Autodesk Fusion 360 part; units mm, degrees
(part 4 of 18)
  line L2686 (171.4183, -55.0432) -> (170.8263, -55.4974)
  line L2687 (174.8684, -55.4974) -> (174.2764, -55.0432)
  line L2688 (173.5871, -54.7577) -> (172.8473, -54.6603)
  line L2689 (174.2764, -55.0432) -> (173.5871, -54.7577)
  line L2690 (172.1076, -54.7577) -> (171.4183, -55.0432)
  line L2691 (170.3721, -58.9475) -> (170.8263, -59.5394)
  line L2692 (175.7055, -57.5184) -> (175.6081, -56.7787)
  line L2693 (175.6081, -56.7787) -> (175.3226, -56.0893)
  line L2694 (174.8684, -59.5394) -> (175.3226, -58.9475)
  line L2695 (172.8473, -54.6603) -> (172.1076, -54.7577)
  line L2696 (175.3226, -58.9475) -> (175.6081, -58.2582)
  line L2697 (170.0866, -58.2582) -> (170.3721, -58.9475)
  line L2698 (172.3659, -83.7435) -> (172.8473, -83.8393)
  line L2699 (173.737, -81.6915) -> (173.3288, -81.4188)
  line L2700 (173.3288, -81.4188) -> (172.8473, -81.323)
  line L2701 (173.3288, -83.7435) -> (173.737, -83.4708)
  line L2702 (173.737, -83.4708) -> (174.0097, -83.0626)
  line L2703 (172.8473, -81.323) -> (172.3659, -81.4188)
  line L2704 (171.9577, -83.4708) -> (172.3659, -83.7435)
  line L2705 (174.0097, -83.0626) -> (174.1055, -82.5812)
  line L2706 (172.3659, -81.4188) -> (171.9577, -81.6915)
  line L2707 (174.1055, -82.5812) -> (174.0097, -82.0997)
  line L2708 (171.5892, -82.5812) -> (171.685, -83.0626)
  line L2709 (171.685, -82.0997) -> (171.5892, -82.5812)
  line L2710 (172.8473, -83.8393) -> (173.3288, -83.7435)
  line L2711 (171.9577, -81.6915) -> (171.685, -82.0997)
  line L2712 (171.685, -83.0626) -> (171.9577, -83.4708)
  line L2713 (174.0097, -82.0997) -> (173.737, -81.6915)
  line L2714 (172.3659, -64.6808) -> (172.8473, -64.7766)
  line L2715 (171.5892, -63.5184) -> (171.685, -63.9999)
  line L2716 (171.9577, -64.4081) -> (172.3659, -64.6808)
  line L2717 (174.0097, -63.9999) -> (174.1055, -63.5184)
  line L2718 (171.9577, -62.6288) -> (171.685, -63.037)
  line L2719 (173.737, -64.4081) -> (174.0097, -63.9999)
  line L2720 (172.8473, -62.2603) -> (172.3659, -62.3561)
  line L2721 (173.3288, -64.6808) -> (173.737, -64.4081)
  line L2722 (171.685, -63.9999) -> (171.9577, -64.4081)
  line L2723 (173.737, -62.6288) -> (173.3288, -62.3561)
  line L2724 (172.8473, -64.7766) -> (173.3288, -64.6808)
  line L2725 (171.685, -63.037) -> (171.5892, -63.5184)
  line L2726 (174.0097, -63.037) -> (173.737, -62.6288)
  line L2727 (172.3659, -62.3561) -> (171.9577, -62.6288)
  line L2728 (173.3288, -62.3561) -> (172.8473, -62.2603)
  line L2729 (174.1055, -63.5184) -> (174.0097, -63.037)
  line L2730 (174.1055, -25.4057) -> (174.0097, -24.9242)
  line L2731 (171.9577, -24.516) -> (171.685, -24.9242)
  line L2732 (173.737, -24.516) -> (173.3288, -24.2433)
  line L2733 (172.8473, -24.1475) -> (172.3659, -24.2433)
  line L2734 (171.5892, -25.4057) -> (171.685, -25.8871)
  line L2735 (173.737, -26.2953) -> (174.0097, -25.8871)
  line L2736 (174.0097, -25.8871) -> (174.1055, -25.4057)
  line L2737 (172.8473, -26.6638) -> (173.3288, -26.568)
  line L2738 (174.0097, -24.9242) -> (173.737, -24.516)
  line L2739 (173.3288, -26.568) -> (173.737, -26.2953)
  line L2740 (171.9577, -26.2953) -> (172.3659, -26.568)
  line L2741 (173.3288, -24.2433) -> (172.8473, -24.1475)
  line L2742 (172.3659, -26.568) -> (172.8473, -26.6638)
  line L2743 (171.685, -24.9242) -> (171.5892, -25.4057)
  line L2744 (171.685, -25.8871) -> (171.9577, -26.2953)
  line L2745 (172.3659, -24.2433) -> (171.9577, -24.516)
  line L2746 (171.9577, -45.3453) -> (172.3659, -45.6181)
  line L2747 (174.1055, -44.4557) -> (174.0097, -43.9742)
  line L2748 (174.0097, -44.9372) -> (174.1055, -44.4557)
  line L2749 (173.3288, -43.2933) -> (172.8473, -43.1975)
  line L2750 (173.737, -43.566) -> (173.3288, -43.2933)
  line L2751 (173.737, -45.3453) -> (174.0097, -44.9372)
  line L2752 (172.8473, -43.1975) -> (172.3659, -43.2933)
  line L2753 (172.8473, -45.7138) -> (173.3288, -45.6181)
  line L2754 (171.685, -43.9742) -> (171.5892, -44.4557)
  line L2755 (173.3288, -45.6181) -> (173.737, -45.3453)
  line L2756 (172.3659, -43.2933) -> (171.9577, -43.566)
  line L2757 (172.3659, -45.6181) -> (172.8473, -45.7138)
  line L2758 (171.9577, -43.566) -> (171.685, -43.9742)
  line L2759 (174.0097, -43.9742) -> (173.737, -43.566)
  line L2760 (171.685, -44.9372) -> (171.9577, -45.3453)
  line L2761 (171.5892, -44.4557) -> (171.685, -44.9372)
  line L2762 (189.8764, -21.4267) -> (190.4683, -21.8809)
  line L2763 (189.8764, -17.3846) -> (189.4222, -17.9766)
  line L2764 (189.4222, -20.8347) -> (189.8764, -21.4267)
  line L2765 (193.9184, -17.3846) -> (193.3265, -16.9304)
  line L2766 (191.8974, -16.5475) -> (191.1576, -16.6449)
  line L2767 (189.1366, -20.1454) -> (189.4222, -20.8347)
  line L2768 (191.8974, -22.2638) -> (192.6371, -22.1664)
  line L2769 (193.3265, -16.9304) -> (192.6371, -16.6449)
  line L2770 (194.3726, -17.9766) -> (193.9184, -17.3846)
  line L2771 (189.4222, -17.9766) -> (189.1366, -18.6659)
  line L2772 (194.6581, -18.6659) -> (194.3726, -17.9766)
  line L2773 (194.6581, -20.1454) -> (194.7555, -19.4056)
  line L2774 (193.9184, -21.4267) -> (194.3726, -20.8347)
  line L2775 (191.1576, -22.1664) -> (191.8974, -22.2638)
  line L2776 (194.3726, -20.8347) -> (194.6581, -20.1454)
  line L2777 (190.4683, -21.8809) -> (191.1576, -22.1664)
  line L2778 (193.3265, -21.8809) -> (193.9184, -21.4267)
  line L2779 (194.7555, -19.4056) -> (194.6581, -18.6659)
  line L2780 (190.4683, -16.9304) -> (189.8764, -17.3846)
  line L2781 (192.6371, -16.6449) -> (191.8974, -16.5475)
  line L2782 (191.1576, -16.6449) -> (190.4683, -16.9304)
  line L2783 (192.6371, -22.1664) -> (193.3265, -21.8809)
  line L2784 (189.1366, -18.6659) -> (189.0392, -19.4056)
  line L2785 (189.0392, -19.4056) -> (189.1366, -20.1454)
  line L2786 (189.4222, -78.0102) -> (189.8764, -78.6022)
  line L2787 (192.6371, -79.3419) -> (193.3265, -79.0564)
  line L2788 (192.6371, -73.8204) -> (191.8974, -73.723)
  line L2789 (193.3265, -74.1059) -> (192.6371, -73.8204)
  line L2790 (191.1576, -79.3419) -> (191.8974, -79.4393)
  line L2791 (194.6581, -75.8414) -> (194.3726, -75.1521)
  line L2792 (194.6581, -77.3209) -> (194.7555, -76.5812)
  line L2793 (190.4683, -74.1059) -> (189.8764, -74.5601)
  line L2794 (191.8974, -79.4393) -> (192.6371, -79.3419)
  line L2795 (191.8974, -73.723) -> (191.1576, -73.8204)
  line L2796 (189.1366, -75.8414) -> (189.0392, -76.5812)
  line L2797 (189.0392, -76.5812) -> (189.1366, -77.3209)
  line L2798 (194.7555, -76.5812) -> (194.6581, -75.8414)
  line L2799 (194.3726, -78.0102) -> (194.6581, -77.3209)
  line L2800 (189.1366, -77.3209) -> (189.4222, -78.0102)
  line L2801 (193.9184, -74.5601) -> (193.3265, -74.1059)
  line L2802 (193.3265, -79.0564) -> (193.9184, -78.6022)
  line L2803 (189.4222, -75.1521) -> (189.1366, -75.8414)
  line L2804 (190.4683, -79.0564) -> (191.1576, -79.3419)
  line L2805 (191.1576, -73.8204) -> (190.4683, -74.1059)
  line L2806 (189.8764, -78.6022) -> (190.4683, -79.0564)
  line L2807 (193.9184, -78.6022) -> (194.3726, -78.0102)
  line L2808 (194.3726, -75.1521) -> (193.9184, -74.5601)
  line L2809 (189.8764, -74.5601) -> (189.4222, -75.1521)
  line L2810 (194.7555, -38.4557) -> (194.6581, -37.7159)
  line L2811 (191.1576, -35.6949) -> (190.4683, -35.9805)
  line L2812 (189.1366, -39.1954) -> (189.4222, -39.8847)
  line L2813 (189.4222, -37.0266) -> (189.1366, -37.7159)
  line L2814 (193.9184, -36.4347) -> (193.3265, -35.9805)
  line L2815 (193.3265, -35.9805) -> (192.6371, -35.6949)
  line L2816 (194.6581, -37.7159) -> (194.3726, -37.0266)
  line L2817 (192.6371, -35.6949) -> (191.8974, -35.5975)
  line L2818 (189.1366, -37.7159) -> (189.0392, -38.4557)
  line L2819 (190.4683, -35.9805) -> (189.8764, -36.4347)
  line L2820 (189.8764, -36.4347) -> (189.4222, -37.0266)
  line L2821 (194.3726, -37.0266) -> (193.9184, -36.4347)
  line L2822 (189.8764, -40.4767) -> (190.4683, -40.9309)
  line L2823 (191.1576, -41.2164) -> (191.8974, -41.3138)
  line L2824 (190.4683, -40.9309) -> (191.1576, -41.2164)
  line L2825 (193.3265, -40.9309) -> (193.9184, -40.4767)
  line L2826 (193.9184, -40.4767) -> (194.3726, -39.8847)
  line L2827 (194.3726, -39.8847) -> (194.6581, -39.1954)
  line L2828 (191.8974, -41.3138) -> (192.6371, -41.2164)
  line L2829 (191.8974, -35.5975) -> (191.1576, -35.6949)
  line L2830 (194.6581, -39.1954) -> (194.7555, -38.4557)
  line L2831 (192.6371, -41.2164) -> (193.3265, -40.9309)
  line L2832 (189.0392, -38.4557) -> (189.1366, -39.1954)
  line L2833 (189.4222, -39.8847) -> (189.8764, -40.4767)
  line L2834 (189.1366, -58.2582) -> (189.4222, -58.9475)
  line L2835 (189.0392, -57.5184) -> (189.1366, -58.2582)
  line L2836 (190.4683, -55.0432) -> (189.8764, -55.4974)
  line L2837 (190.4683, -59.9936) -> (191.1576, -60.2792)
  line L2838 (191.1576, -54.7577) -> (190.4683, -55.0432)
  line L2839 (191.8974, -60.3766) -> (192.6371, -60.2792)
  line L2840 (192.6371, -54.7577) -> (191.8974, -54.6603)
  line L2841 (192.6371, -60.2792) -> (193.3265, -59.9936)
  line L2842 (191.8974, -54.6603) -> (191.1576, -54.7577)
  line L2843 (194.3726, -58.9475) -> (194.6581, -58.2582)
  line L2844 (189.1366, -56.7787) -> (189.0392, -57.5184)
  line L2845 (193.3265, -55.0432) -> (192.6371, -54.7577)
  line L2846 (191.1576, -60.2792) -> (191.8974, -60.3766)
  line L2847 (194.3726, -56.0893) -> (193.9184, -55.4974)
  line L2848 (189.4222, -58.9475) -> (189.8764, -59.5394)
  line L2849 (193.3265, -59.9936) -> (193.9184, -59.5394)
  line L2850 (189.4222, -56.0893) -> (189.1366, -56.7787)
  line L2851 (194.7555, -57.5184) -> (194.6581, -56.7787)
  line L2852 (189.8764, -59.5394) -> (190.4683, -59.9936)
  line L2853 (194.6581, -56.7787) -> (194.3726, -56.0893)
  line L2854 (189.8764, -55.4974) -> (189.4222, -56.0893)
  line L2855 (193.9184, -59.5394) -> (194.3726, -58.9475)
  line L2856 (193.9184, -55.4974) -> (193.3265, -55.0432)
  line L2857 (194.6581, -58.2582) -> (194.7555, -57.5184)
  line L2858 (193.0598, -82.0997) -> (192.787, -81.6915)
  line L2859 (193.0598, -83.0626) -> (193.1555, -82.5812)
  line L2860 (191.0077, -83.4708) -> (191.4159, -83.7435)
  line L2861 (191.8974, -81.323) -> (191.4159, -81.4188)
  line L2862 (192.3789, -83.7435) -> (192.787, -83.4708)
  line L2863 (192.3789, -81.4188) -> (191.8974, -81.323)
  line L2864 (191.4159, -81.4188) -> (191.0077, -81.6915)
  line L2865 (190.735, -82.0997) -> (190.6392, -82.5812)
  line L2866 (191.0077, -81.6915) -> (190.735, -82.0997)
  line L2867 (193.1555, -82.5812) -> (193.0598, -82.0997)
  line L2868 (192.787, -81.6915) -> (192.3789, -81.4188)
  line L2869 (192.787, -83.4708) -> (193.0598, -83.0626)
  line L2870 (191.8974, -83.8393) -> (192.3789, -83.7435)
  line L2871 (191.4159, -83.7435) -> (191.8974, -83.8393)
  line L2872 (190.6392, -82.5812) -> (190.735, -83.0626)
  line L2873 (190.735, -83.0626) -> (191.0077, -83.4708)
  line L2874 (192.3789, -64.6808) -> (192.787, -64.4081)
  line L2875 (192.3789, -62.3561) -> (191.8974, -62.2603)
  line L2876 (191.4159, -62.3561) -> (191.0077, -62.6288)
  line L2877 (190.735, -63.9999) -> (191.0077, -64.4081)
  line L2878 (193.0598, -63.9999) -> (193.1555, -63.5184)
  line L2879 (191.4159, -64.6808) -> (191.8974, -64.7766)
  line L2880 (192.787, -62.6288) -> (192.3789, -62.3561)
  line L2881 (193.0598, -63.037) -> (192.787, -62.6288)
  line L2882 (193.1555, -63.5184) -> (193.0598, -63.037)
  line L2883 (191.0077, -62.6288) -> (190.735, -63.037)
  line L2884 (191.8974, -64.7766) -> (192.3789, -64.6808)
  line L2885 (191.8974, -62.2603) -> (191.4159, -62.3561)
  line L2886 (190.735, -63.037) -> (190.6392, -63.5184)
  line L2887 (192.787, -64.4081) -> (193.0598, -63.9999)
  line L2888 (191.0077, -64.4081) -> (191.4159, -64.6808)
  line L2889 (190.6392, -63.5184) -> (190.735, -63.9999)
  line L2890 (191.4159, -26.568) -> (191.8974, -26.6638)
  line L2891 (192.3789, -24.2433) -> (191.8974, -24.1475)
  line L2892 (191.8974, -24.1475) -> (191.4159, -24.2433)
  line L2893 (192.3789, -26.568) -> (192.787, -26.2953)
  line L2894 (190.735, -25.8871) -> (191.0077, -26.2953)
  line L2895 (191.4159, -24.2433) -> (191.0077, -24.516)
  line L2896 (190.735, -24.9242) -> (190.6392, -25.4057)
  line L2897 (191.8974, -26.6638) -> (192.3789, -26.568)
  line L2898 (193.0598, -24.9242) -> (192.787, -24.516)
  line L2899 (192.787, -26.2953) -> (193.0598, -25.8871)
  line L2900 (193.0598, -25.8871) -> (193.1555, -25.4057)
  line L2901 (193.1555, -25.4057) -> (193.0598, -24.9242)
  line L2902 (192.787, -24.516) -> (192.3789, -24.2433)
  line L2903 (191.0077, -26.2953) -> (191.4159, -26.568)
  line L2904 (190.6392, -25.4057) -> (190.735, -25.8871)
  line L2905 (191.0077, -24.516) -> (190.735, -24.9242)
  line L2906 (193.1555, -44.4557) -> (193.0598, -43.9742)
  line L2907 (191.4159, -45.6181) -> (191.8974, -45.7138)
  line L2908 (192.3789, -45.6181) -> (192.787, -45.3453)
  line L2909 (192.3789, -43.2933) -> (191.8974, -43.1975)
  line L2910 (190.735, -44.9372) -> (191.0077, -45.3453)
  line L2911 (191.8974, -45.7138) -> (192.3789, -45.6181)
  line L2912 (193.0598, -44.9372) -> (193.1555, -44.4557)
  line L2913 (192.787, -45.3453) -> (193.0598, -44.9372)
  line L2914 (191.8974, -43.1975) -> (191.4159, -43.2933)
  line L2915 (192.787, -43.566) -> (192.3789, -43.2933)
  line L2916 (193.0598, -43.9742) -> (192.787, -43.566)
  line L2917 (191.0077, -43.566) -> (190.735, -43.9742)
  line L2918 (190.735, -43.9742) -> (190.6392, -44.4557)
  line L2919 (190.6392, -44.4557) -> (190.735, -44.9372)
  line L2920 (191.0077, -45.3453) -> (191.4159, -45.6181)
  line L2921 (191.4159, -43.2933) -> (191.0077, -43.566)
  line L2922 (207.8352, -8.2676) -> (207.7686, -8.6245)
  line L2923 (208.4289, -10.8261) -> (208.7781, -10.7267)
  line L2924 (207.7686, -8.6245) -> (207.8999, -8.9629)
  line L2925 (207.8999, -8.9629) -> (207.7811, -9.2209)
  line L2926 (209.0892, -8.6245) -> (209.0226, -8.2676)
  line L2927 (208.4289, -7.8999) -> (208.0797, -7.9992)
  line L2928 (209.0892, -10.1014) -> (208.9578, -9.7629)
  line L2929 (208.0797, -10.7267) -> (208.4289, -10.8261)
  line L2930 (209.0767, -9.2209) -> (208.9579, -8.9629)
  line L2931 (207.8351, -10.4583) -> (208.0797, -10.7267)
  line L2932 (208.9579, -8.9629) -> (209.0892, -8.6245)
  line L2933 (209.0226, -8.2676) -> (208.7781, -7.9992)
  line L2934 (208.0797, -7.9992) -> (207.8352, -8.2676)
  line L2935 (208.7781, -7.9992) -> (208.4289, -7.8999)
  line L2936 (208.9578, -9.7629) -> (209.0766, -9.5049)
  line L2937 (209.0766, -9.5049) -> (209.0767, -9.2209)
  line L2938 (208.7781, -10.7267) -> (209.0226, -10.4583)
  line L2939 (207.7686, -10.1014) -> (207.8351, -10.4583)
  line L2940 (207.9, -9.7629) -> (207.7686, -10.1014)
  line L2941 (207.7811, -9.2209) -> (207.7811, -9.5049)
  line L2942 (207.7811, -9.5049) -> (207.9, -9.7629)
  line L2943 (209.0226, -10.4583) -> (209.0892, -10.1014)
  line L2944 (208.0893, -76.5812) -> (208.1867, -77.3209)
  line L2945 (211.6872, -73.8204) -> (210.9474, -73.723)
  line L2946 (211.6872, -79.3419) -> (212.3765, -79.0564)
  line L2947 (210.9474, -73.723) -> (210.2077, -73.8204)
  line L2948 (213.7082, -75.8414) -> (213.4226, -75.1521)
  line L2949 (213.8056, -76.5812) -> (213.7082, -75.8414)
  line L2950 (209.5183, -74.1059) -> (208.9264, -74.5601)
  line L2951 (213.4226, -75.1521) -> (212.9684, -74.5601)
  line L2952 (208.9264, -74.5601) -> (208.4722, -75.1521)
  line L2953 (212.9684, -78.6022) -> (213.4226, -78.0102)
  line L2954 (208.1867, -75.8414) -> (208.0893, -76.5812)
  line L2955 (212.3765, -79.0564) -> (212.9684, -78.6022)
  line L2956 (210.9474, -79.4393) -> (211.6872, -79.3419)
  line L2957 (208.9264, -78.6022) -> (209.5183, -79.0564)
  line L2958 (208.4722, -78.0102) -> (208.9264, -78.6022)
  line L2959 (210.2077, -79.3419) -> (210.9474, -79.4393)
  line L2960 (212.3765, -74.1059) -> (211.6872, -73.8204)
  line L2961 (213.4226, -78.0102) -> (213.7082, -77.3209)
  line L2962 (208.1867, -77.3209) -> (208.4722, -78.0102)
  line L2963 (213.7082, -77.3209) -> (213.8056, -76.5812)
  line L2964 (209.5183, -79.0564) -> (210.2077, -79.3419)
  line L2965 (208.4722, -75.1521) -> (208.1867, -75.8414)
  line L2966 (212.9684, -74.5601) -> (212.3765, -74.1059)
  line L2967 (210.2077, -73.8204) -> (209.5183, -74.1059)
  line L2968 (216.799, -60.0016) -> (217.1027, -59.9279)
  line L2969 (210.1483, -15.278) -> (210.164, -15.5734)
  line L2970 (215.6109, -79.8483) -> (215.3395, -79.4399)
  line L2971 (211.1455, -12.7014) -> (210.8777, -12.5495)
  line L2972 (213.5586, -81.2176) -> (213.9665, -81.4897)
  line L2973 (213.1498, -21.2274) -> (213.5446, -20.5988)
  line L2974 (213.9408, -10.8643) -> (213.7416, -10.6234)
  line L2975 (212.6905, -11.2642) -> (212.8134, -11.5516)
  line L2976 (213.5559, -41.3139) -> (213.2846, -41.7214)
  line L2977 (217.9096, -13.4521) -> (218.0606, -13.1871)
  line L2978 (208.2794, -20.4305) -> (208.6333, -21.0831)
  line L2979 (210.4841, -14.8092) -> (210.2625, -15.0052)
  line L2980 (217.9096, -14.6609) -> (217.9096, -13.4521)
  line L2981 (210.1086, -13.4992) -> (209.8976, -13.6892)
  line L2982 (216.9393, -13.4521) -> (216.9393, -14.1014)
  line L2983 (216.2203, -18.2275) -> (214.8817, -16.8888)
  line L2984 (217.8008, -15.659) -> (217.9939, -15.4528)
  line L2985 (212.8134, -11.5516) -> (213.0543, -11.7508)
  line L2986 (214.8817, -16.8888) -> (215.1771, -16.7608)
  line L2987 (208.7163, -17.6193) -> (208.3315, -18.2542)
  line L2988 (213.9623, -41.0408) -> (213.5559, -41.3139)
  line L2989 (214.7969, -15.5718) -> (212.0686, -12.8435)
  line L2990 (213.7416, -10.6234) -> (213.4542, -10.5006)
  line L2991 (217.2571, -58.859) -> (217.2571, -15.7547)
  line L2992 (216.295, -18.3257) -> (216.2203, -18.2275)
  line L2993 (217.9554, -12.6027) -> (217.7213, -12.4071)
  line L2994 (213.1893, -42.2017) -> (213.2846, -42.6819)
  line L2995 (209.2516, -17.105) -> (208.7163, -17.6193)
  line L2996 (213.9665, -81.4897) -> (214.4474, -81.5853)
  line L2997 (210.5476, -16.0039) -> (210.8392, -16.0534)
  line L2998 (209.9013, -16.7458) -> (209.2516, -17.105)
  line L2999 (213.9623, -62.4253) -> (213.9623, -79.1663)
  line L3000 (216.3408, -18.4403) -> (216.295, -18.3257)
  line L3001 (211.2279, -22.25) -> (211.951, -22.0818)
  line L3002 (210.4859, -22.2263) -> (211.2279, -22.25)
  line L3003 (213.7643, -19.8896) -> (213.7643, -22.0951)
  line L3004 (214.4474, -81.5853) -> (214.9284, -81.4897)
  line L3005 (217.4258, -59.1221) -> (217.2571, -58.859)
  line L3006 (211.7256, -12.7014) -> (211.1455, -12.7014)
  line L3007 (218.0537, -14.9039) -> (217.9096, -14.6609)
  line L3008 (210.6215, -16.5661) -> (209.9013, -16.7458)
  line L3009 (213.2857, -80.8102) -> (213.5586, -81.2176)
  line L3010 (217.1027, -59.9279) -> (217.339, -59.7234)
  line L3011 (213.3151, -23.7) -> (213.5827, -24.0655)
  line L3012 (211.951, -22.0818) -> (212.6063, -21.7331)
  line L3013 (215.1063, -15.661) -> (214.7969, -15.5718)
  line L3014 (213.5559, -62.1522) -> (213.9623, -62.4253)
  line L3015 (208.3315, -18.2542) -> (208.1232, -18.9667)
  line L3016 (213.3596, -11.8175) -> (216.3408, -14.7987)
  line L3017 (209.8976, -13.6892) -> (209.7854, -13.95)
  line L3018 (213.2846, -61.7447) -> (213.5559, -62.1522)
  line L3019 (210.8392, -16.0534) -> (211.3638, -16.578)
  line L3020 (213.9623, -43.3625) -> (213.9623, -60.1036)
  line L3021 (210.0304, -13.2013) -> (210.1086, -13.4992)
  line L3022 (214.0075, -11.1696) -> (213.9408, -10.8643)
  line L3023 (217.5394, -15.7661) -> (217.8008, -15.659)
  line L3024 (215.2794, -43.1455) -> (215.5383, -42.8285)
  line L3025 (215.6818, -42.4453) -> (216.0297, -42.4675)
  line L3026 (216.3408, -42.31) -> (216.3408, -58.859)
  line L3027 (216.0297, -42.4675) -> (216.3408, -42.31)
  line L3028 (216.3408, -58.859) -> (216.1721, -59.1221)
  line L3029 (216.1426, -59.4333) -> (216.2589, -59.7234)
  line L3030 (216.1721, -59.1221) -> (216.1426, -59.4333)
  line L3031 (216.2589, -59.7234) -> (216.4952, -59.9279)
  line L3032 (216.4952, -59.9279) -> (216.799, -60.0016)
  line L3033 (214.9326, -60.1036) -> (214.9326, -43.3625)
  line L3034 (215.3389, -60.3767) -> (214.9326, -60.1036)
  line L3035 (215.5383, -42.8285) -> (215.6818, -42.4453)
  line L3036 (214.9326, -43.3625) -> (215.2794, -43.1455)
  line L3037 (215.1771, -16.7608) -> (215.3774, -16.5087)
  line L3038 (213.5827, -24.0655) -> (213.9623, -24.3125)
  line L3039 (218.0771, -12.8825) -> (217.9554, -12.6027)
  line L3040 (213.5446, -20.5988) -> (213.7643, -19.8896)
  line L3041 (216.3408, -14.7987) -> (216.3408, -18.4403)
  line L3042 (210.4131, -14.7383) -> (210.4841, -14.8092)
  line L3043 (208.6333, -21.0831) -> (209.1433, -21.6225)
  line L3044 (213.284, -79.8483) -> (213.1893, -80.3294)
  line L3045 (213.4344, -22.4055) -> (213.2358, -22.8125)
  line L3046 (212.6063, -21.7331) -> (213.1498, -21.2274)
  line L3047 (213.9623, -24.3125) -> (213.9623, -41.0408)
  line L3048 (217.339, -59.7234) -> (217.4553, -59.4333)
  line L3049 (216.7882, -13.1871) -> (216.9393, -13.4521)
  line L3050 (209.1433, -21.6225) -> (209.7751, -22.0123)
  line L3051 (218.0606, -13.1871) -> (218.0771, -12.8825)
  line L3052 (217.9939, -15.4528) -> (218.0837, -15.1849)
  line L3053 (213.7643, -22.0951) -> (213.4344, -22.4055)
  line L3054 (216.9393, -14.1014) -> (214.0075, -11.1696)
  line L3055 (210.2891, -12.661) -> (210.0953, -12.9003)
  line L3056 (217.7213, -12.4071) -> (217.4244, -12.3369)
  line L3057 (217.1275, -12.4071) -> (216.8935, -12.6027)
  line L3058 (212.7129, -10.9525) -> (212.6905, -11.2642)
  line L3059 (218.0837, -15.1849) -> (218.0537, -14.9039)
  line L3060 (213.5559, -60.3767) -> (213.2846, -60.7842)
  line L3061 (212.0686, -12.8435) -> (211.9112, -12.7384)
  line L3062 (213.1943, -23.2635) -> (213.3151, -23.7)
  line L3063 (215.3373, -15.8853) -> (215.1063, -15.661)
  line L3064 (213.4542, -10.5006) -> (213.1425, -10.5229)
  line L3065 (213.2846, -41.7214) -> (213.1893, -42.2017)
  line L3066 (213.1893, -61.2644) -> (213.2846, -61.7447)
  line L3067 (208.1054, -19.7088) -> (208.2794, -20.4305)
  line L3068 (215.7056, -61.2644) -> (215.6103, -60.7842)
  line L3069 (215.3395, -79.4399) -> (214.9326, -79.1663)
  line L3070 (215.3389, -62.1522) -> (215.6103, -61.7447)
  line L3071 (215.6103, -60.7842) -> (215.3389, -60.3767)
  line L3072 (215.7056, -80.3294) -> (215.6109, -79.8483)
  line L3073 (214.9326, -79.1663) -> (214.9326, -62.4253)
  line L3074 (215.6103, -61.7447) -> (215.7056, -61.2644)
  line L3075 (213.2846, -42.6819) -> (213.5559, -43.0894)
  line L3076 (213.5554, -79.4399) -> (213.284, -79.8483)
  line L3077 (210.5701, -12.535) -> (210.2891, -12.661)
  line L3078 (213.5559, -43.0894) -> (213.9623, -43.3625)
  line L3079 (214.9284, -81.4897) -> (215.3363, -81.2176)
  line L3080 (209.9178, -14.4887) -> (210.1381, -14.6678)
  line L3081 (209.7751, -22.0123) -> (210.4859, -22.2263)
  line L3082 (215.6091, -80.8102) -> (215.7056, -80.3294)
  line L3083 (213.2846, -60.7842) -> (213.1893, -61.2644)
  line L3084 (211.9112, -12.7384) -> (211.7256, -12.7014)
  line L3085 (209.7854, -13.95) -> (209.7925, -14.2338)
  line L3086 (216.7718, -12.8825) -> (216.7882, -13.1871)
  line L3087 (213.1893, -80.3294) -> (213.2857, -80.8102)
  line L3088 (217.4244, -12.3369) -> (217.1275, -12.4071)
  line L3089 (213.9623, -60.1036) -> (213.5559, -60.3767)
  line L3090 (213.9623, -79.1663) -> (213.5554, -79.4399)
  line L3091 (210.2625, -15.0052) -> (210.1483, -15.278)
  line L3092 (213.2358, -22.8125) -> (213.1943, -23.2635)
  line L3093 (208.1232, -18.9667) -> (208.1054, -19.7088)
  line L3094 (215.3774, -16.5087) -> (215.4353, -16.192)
  line L3095 (217.4553, -59.4333) -> (217.4258, -59.1221)
  line L3096 (210.0953, -12.9003) -> (210.0304, -13.2013)
  line L3097 (215.3363, -81.2176) -> (215.6091, -80.8102)
  line L3098 (216.8935, -12.6027) -> (216.7718, -12.8825)
  line L3099 (210.3066, -15.8325) -> (210.5476, -16.0039)
  line L3100 (215.4353, -16.192) -> (215.3373, -15.8853)
  line L3101 (210.8777, -12.5495) -> (210.5701, -12.535)
  line L3102 (210.1381, -14.6678) -> (210.4131, -14.7383)
  line L3103 (213.1425, -10.5229) -> (212.8756, -10.6856)
  line L3104 (212.8756, -10.6856) -> (212.7129, -10.9525)
  line L3105 (210.164, -15.5734) -> (210.3066, -15.8325)
  line L3106 (213.0543, -11.7508) -> (213.3596, -11.8175)
  line L3107 (209.7925, -14.2338) -> (209.9178, -14.4887)
  line L3108 (217.2571, -15.7547) -> (217.5394, -15.7661)
  line L3109 (214.9326, -62.4253) -> (215.3389, -62.1522)
  line L3110 (211.3638, -16.578) -> (210.6215, -16.5661)
  line L3111 (212.9684, -40.4767) -> (213.4226, -39.8847)
  line L3112 (213.8056, -38.4557) -> (213.7082, -37.7159)
  line L3113 (208.0893, -38.4557) -> (208.1867, -39.1954)
  line L3114 (212.9684, -36.4347) -> (212.3765, -35.9805)
  line L3115 (211.6872, -35.6949) -> (210.9474, -35.5975)
  line L3116 (208.9264, -40.4767) -> (209.5183, -40.9309)
  line L3117 (208.1867, -37.7159) -> (208.0893, -38.4557)
  line L3118 (213.4226, -37.0266) -> (212.9684, -36.4347)
  line L3119 (213.4226, -39.8847) -> (213.7082, -39.1954)
  line L3120 (208.1867, -39.1954) -> (208.4722, -39.8847)
  line L3121 (210.9474, -35.5975) -> (210.2077, -35.6949)
  line L3122 (210.2077, -41.2164) -> (210.9474, -41.3138)
  line L3123 (208.9264, -36.4347) -> (208.4722, -37.0266)
  line L3124 (210.9474, -41.3138) -> (211.6872, -41.2164)
  line L3125 (209.5183, -40.9309) -> (210.2077, -41.2164)
  line L3126 (210.2077, -35.6949) -> (209.5183, -35.9805)
  line L3127 (213.7082, -39.1954) -> (213.8056, -38.4557)
  line L3128 (209.5183, -35.9805) -> (208.9264, -36.4347)
  line L3129 (212.3765, -35.9805) -> (211.6872, -35.6949)
  line L3130 (212.3765, -40.9309) -> (212.9684, -40.4767)
  line L3131 (208.4722, -37.0266) -> (208.1867, -37.7159)
  line L3132 (213.7082, -37.7159) -> (213.4226, -37.0266)
  line L3133 (208.4722, -39.8847) -> (208.9264, -40.4767)
  line L3134 (211.6872, -41.2164) -> (212.3765, -40.9309)
  line L3135 (213.7082, -58.2582) -> (213.8056, -57.5184)
  line L3136 (211.6872, -54.7577) -> (210.9474, -54.6603)
  line L3137 (208.1867, -56.7787) -> (208.0893, -57.5184)
  line L3138 (208.9264, -59.5394) -> (209.5183, -59.9936)
  line L3139 (208.4722, -58.9475) -> (208.9264, -59.5394)
  line L3140 (213.7082, -56.7787) -> (213.4226, -56.0893)
  line L3141 (208.4722, -56.0893) -> (208.1867, -56.7787)
  line L3142 (212.3765, -59.9936) -> (212.9684, -59.5394)
  line L3143 (212.3765, -55.0432) -> (211.6872, -54.7577)
  line L3144 (208.1867, -58.2582) -> (208.4722, -58.9475)
  line L3145 (210.2077, -60.2792) -> (210.9474, -60.3766)
  line L3146 (213.4226, -56.0893) -> (212.9684, -55.4974)
  line L3147 (212.9684, -55.4974) -> (212.3765, -55.0432)
  line L3148 (211.6872, -60.2792) -> (212.3765, -59.9936)
  line L3149 (210.2077, -54.7577) -> (209.5183, -55.0432)
  line L3150 (213.4226, -58.9475) -> (213.7082, -58.2582)
  line L3151 (208.0893, -57.5184) -> (208.1867, -58.2582)
  line L3152 (213.8056, -57.5184) -> (213.7082, -56.7787)
  line L3153 (208.9264, -55.4974) -> (208.4722, -56.0893)
  line L3154 (209.5183, -55.0432) -> (208.9264, -55.4974)
  line L3155 (210.9474, -54.6603) -> (210.2077, -54.7577)
  line L3156 (209.5183, -59.9936) -> (210.2077, -60.2792)
  line L3157 (210.9474, -60.3766) -> (211.6872, -60.2792)
  line L3158 (212.9684, -59.5394) -> (213.4226, -58.9475)
  line L3159 (210.9474, -81.323) -> (210.466, -81.4188)
  line L3160 (211.4289, -81.4188) -> (210.9474, -81.323)
  line L3161 (211.4289, -83.7435) -> (211.8371, -83.4708)
  line L3162 (209.6893, -82.5812) -> (209.7851, -83.0626)
  line L3163 (210.9474, -83.8393) -> (211.4289, -83.7435)
  line L3164 (210.466, -81.4188) -> (210.0578, -81.6915)
  line L3165 (209.7851, -82.0997) -> (209.6893, -82.5812)
  line L3166 (212.2056, -82.5812) -> (212.1098, -82.0997)
  line L3167 (210.0578, -81.6915) -> (209.7851, -82.0997)
  line L3168 (211.8371, -83.4708) -> (212.1098, -83.0626)
  line L3169 (212.1098, -82.0997) -> (211.8371, -81.6915)
  line L3170 (209.7851, -83.0626) -> (210.0578, -83.4708)
  line L3171 (212.1098, -83.0626) -> (212.2056, -82.5812)
  line L3172 (210.0578, -83.4708) -> (210.466, -83.7435)
  line L3173 (210.466, -83.7435) -> (210.9474, -83.8393)
  line L3174 (211.8371, -81.6915) -> (211.4289, -81.4188)
  line L3175 (211.4289, -64.6808) -> (211.8371, -64.4081)
  line L3176 (211.4289, -62.3561) -> (210.9474, -62.2603)
  line L3177 (210.9474, -64.7766) -> (211.4289, -64.6808)
  line L3178 (212.2056, -63.5184) -> (212.1098, -63.037)
  line L3179 (210.0578, -64.4081) -> (210.466, -64.6808)
  line L3180 (209.7851, -63.9999) -> (210.0578, -64.4081)
  line L3181 (210.466, -64.6808) -> (210.9474, -64.7766)
  line L3182 (209.7851, -63.037) -> (209.6893, -63.5184)
  line L3183 (212.1098, -63.9999) -> (212.2056, -63.5184)
  line L3184 (211.8371, -62.6288) -> (211.4289, -62.3561)
  line L3185 (210.0578, -62.6288) -> (209.7851, -63.037)
  line L3186 (210.9474, -62.2603) -> (210.466, -62.3561)
  line L3187 (209.6893, -63.5184) -> (209.7851, -63.9999)
  line L3188 (212.1098, -63.037) -> (211.8371, -62.6288)
  line L3189 (211.8371, -64.4081) -> (212.1098, -63.9999)
  line L3190 (210.466, -62.3561) -> (210.0578, -62.6288)
  line L3191 (212.1098, -24.9242) -> (211.8371, -24.516)
  line L3192 (210.0578, -24.516) -> (209.7851, -24.9242)
  line L3193 (212.2056, -25.4057) -> (212.1098, -24.9242)
  line L3194 (210.9474, -24.1475) -> (210.466, -24.2433)
  line L3195 (209.7851, -24.9242) -> (209.6893, -25.4057)
  line L3196 (210.466, -26.568) -> (210.9474, -26.6638)
  line L3197 (211.8371, -26.2953) -> (212.1098, -25.8871)
  line L3198 (212.1098, -25.8871) -> (212.2056, -25.4057)
  line L3199 (211.4289, -26.568) -> (211.8371, -26.2953)
  line L3200 (209.6893, -25.4057) -> (209.7851, -25.8871)
  line L3201 (210.0578, -26.2953) -> (210.466, -26.568)
  line L3202 (211.4289, -24.2433) -> (210.9474, -24.1475)
  line L3203 (210.466, -24.2433) -> (210.0578, -24.516)
  line L3204 (210.9474, -26.6638) -> (211.4289, -26.568)
  line L3205 (209.7851, -25.8871) -> (210.0578, -26.2953)
  line L3206 (211.8371, -24.516) -> (211.4289, -24.2433)
  line L3207 (211.8371, -45.3453) -> (212.1098, -44.9372)
  line L3208 (212.2056, -44.4557) -> (212.1098, -43.9742)
  line L3209 (210.466, -45.6181) -> (210.9474, -45.7138)
  line L3210 (212.1098, -44.9372) -> (212.2056, -44.4557)
  line L3211 (211.4289, -43.2933) -> (210.9474, -43.1975)
  line L3212 (209.7851, -44.9372) -> (210.0578, -45.3453)
  line L3213 (211.4289, -45.6181) -> (211.8371, -45.3453)
  line L3214 (209.7851, -43.9742) -> (209.6893, -44.4557)
  line L3215 (210.9474, -43.1975) -> (210.466, -43.2933)
  line L3216 (211.8371, -43.566) -> (211.4289, -43.2933)
  line L3217 (212.1098, -43.9742) -> (211.8371, -43.566)
  line L3218 (210.0578, -45.3453) -> (210.466, -45.6181)
  line L3219 (209.6893, -44.4557) -> (209.7851, -44.9372)
  line L3220 (210.466, -43.2933) -> (210.0578, -43.566)
  line L3221 (210.9474, -45.7138) -> (211.4289, -45.6181)
  line L3222 (210.0578, -43.566) -> (209.7851, -43.9742)
  line L3223 (180.4463, -4.8901) -> (180.4792, -5.1322)
  line L3224 (180.4747, -3.5648) -> (180.4463, -3.7901)
  line L3225 (177.0589, -5.0311) -> (177.2463, -4.6094)
  line L3226 (177.269, -4.1485) -> (177.124, -3.7104)
  line L3227 (177.2463, -4.6094) -> (177.269, -4.1485)
  line L3228 (180.4792, -5.1322) -> (180.5755, -5.3569)
  line L3229 (180.5581, -3.3537) -> (180.4747, -3.5648)
  line L3230 (176.8308, -3.354) -> (180.5581, -3.3537)
  line L3231 (180.4463, -3.7901) -> (180.4463, -4.8901)
  line L3232 (177.124, -3.7104) -> (176.8308, -3.354)
  line L3233 (176.7321, -5.3569) -> (177.0589, -5.0311)
  line L3234 (180.5755, -5.3569) -> (176.7321, -5.3569)
  line L3235 (189.119, -5.1322) -> (189.2153, -5.3569)
  line L3236 (188.0999, -4.341) -> (188.4228, -4.5083)
  line L3237 (182.2297, -5.1322) -> (182.2626, -4.8901)
  line L3238 (188.7859, -4.4861) -> (189.0861, -4.2808)
  line L3239 (183.2485, -4.341) -> (183.4398, -4.0319)
  line L3240 (189.0861, -4.2808) -> (189.0861, -4.8901)
  line L3241 (183.4455, -3.6683) -> (183.2638, -3.3534)
  line L3242 (182.5628, -4.4862) -> (182.9257, -4.5083)
  line L3243 (182.2626, -4.2811) -> (182.5628, -4.4862)
  line L3244 (187.9086, -4.0316) -> (188.0999, -4.341)
  line L3245 (183.2638, -3.3534) -> (188.0852, -3.353)
  line L3246 (189.2153, -5.3569) -> (182.1334, -5.3569)
  line L3247 (182.9257, -4.5083) -> (183.2485, -4.341)
  line L3248 (187.9032, -3.6679) -> (187.9086, -4.0316)
  line L3249 (182.2626, -4.8901) -> (182.2626, -4.2811)
  line L3250 (182.1334, -5.3569) -> (182.2297, -5.1322)
  line L3251 (189.0861, -4.8901) -> (189.119, -5.1322)
  line L3252 (183.4398, -4.0319) -> (183.4455, -3.6683)
  line L3253 (188.0852, -3.353) -> (187.9032, -3.6679)
  line L3254 (188.4228, -4.5083) -> (188.7859, -4.4861)
  line L3255 (9.6631, -6.3586) -> (9.6631, -6.6177)
  line L3256 (9.6631, -4.5637) -> (9.6631, -4.3046)
  line L3257 (8.7656, -5.4611) -> (8.5065, -5.4611)
  line L3258 (10.5605, -5.4611) -> (10.8196, -5.4611)
  line L3259 (4.1604, 0.039) -> (4.4195, 0.039)
  line L3260 (0.1655, 0.039) -> (-0.0936, 0.039)
  line L3261 (2.1629, -1.1085) -> (2.1629, -1.3676)
  line L3262 (190.5417, -4.3401) -> (190.8008, -4.3401)
  line L3263 (189.4468, -4.3401) -> (189.1877, -4.3401)
  line L3264 (181.9019, -4.3401) -> (182.161, -4.3401)
  line L3265 (180.807, -4.3401) -> (180.5479, -4.3401)
  line L3266 (190.5417, -0.19) -> (190.8008, -0.19)
  line L3267 (189.4468, -0.19) -> (189.1877, -0.19)
  line L3268 (189.9943, 0.7575) -> (189.9943, 1.0166)
  line L3269 (181.9019, -0.19) -> (182.161, -0.19)
  line L3270 (180.807, -0.19) -> (180.5479, -0.19)
  line L3271 (181.3545, 0.7575) -> (181.3545, 1.0166)
  line L3272 (189.9943, -5.4401) -> (189.7193, -5.3664)
  line L3273 (189.518, -3.5151) -> (189.7193, -3.3138)
  line L3274 (189.4443, -3.7901) -> (189.518, -3.5151)
  line L3275 (189.518, -5.1651) -> (189.4443, -4.8901)
  line L3276 (190.5443, -3.7901) -> (190.5443, -4.8901)
  line L3277 (190.2693, -3.3138) -> (190.4706, -3.5151)
  line L3278 (189.7193, -3.3138) -> (189.9943, -3.2401)
  line L3279 (189.4443, -4.8901) -> (189.4443, -3.7901)
  line L3280 (190.4706, -5.1651) -> (190.2693, -5.3664)
  line L3281 (190.5443, -4.8901) -> (190.4706, -5.1651)
  line L3282 (190.2693, -5.3664) -> (189.9943, -5.4401)
  line L3283 (189.9943, -3.2401) -> (190.2693, -3.3138)
  line L3284 (189.7193, -5.3664) -> (189.518, -5.1651)
  line L3285 (190.4706, -3.5151) -> (190.5443, -3.7901)
  line L3286 (181.9045, -4.8901) -> (181.8308, -5.1651)
  line L3287 (180.8045, -4.8901) -> (180.8045, -3.7901)
  line L3288 (181.9045, -3.7901) -> (181.9045, -4.8901)
  line L3289 (180.8045, -3.7901) -> (180.8781, -3.5151)
  line L3290 (181.3545, -5.4401) -> (181.0795, -5.3664)
  line L3291 (181.8308, -5.1651) -> (181.6295, -5.3664)
  line L3292 (181.3545, -3.2401) -> (181.6295, -3.3138)
  line L3293 (180.8781, -5.1651) -> (180.8045, -4.8901)
  line L3294 (181.6295, -3.3138) -> (181.8308, -3.5151)
  line L3295 (181.6295, -5.3664) -> (181.3545, -5.4401)
  line L3296 (181.0795, -3.3138) -> (181.3545, -3.2401)
  line L3297 (180.8781, -3.5151) -> (181.0795, -3.3138)
  line L3298 (181.8308, -3.5151) -> (181.9045, -3.7901)
  line L3299 (181.0795, -5.3664) -> (180.8781, -5.1651)
  line L3300 (189.518, 0.485) -> (189.7193, 0.6863)
  line L3301 (189.4443, -0.59) -> (189.4443, 0.21)
  line L3302 (190.4706, -0.865) -> (190.2693, -1.0663)
  line L3303 (190.4706, 0.485) -> (190.5443, 0.21)
  line L3304 (189.7193, 0.6863) -> (189.9943, 0.76)
  line L3305 (189.518, -0.865) -> (189.4443, -0.59)
  line L3306 (190.2693, 0.6863) -> (190.4706, 0.485)
  line L3307 (190.5443, 0.21) -> (190.5443, -0.59)
  line L3308 (189.4443, 0.21) -> (189.518, 0.485)
  line L3309 (189.9943, 0.76) -> (190.2693, 0.6863)
  line L3310 (190.5443, -0.59) -> (190.4706, -0.865)
  line L3311 (190.2693, -1.0663) -> (189.9943, -1.14)
  line L3312 (189.7193, -1.0663) -> (189.518, -0.865)
  line L3313 (189.9943, -1.14) -> (189.7193, -1.0663)
  line L3314 (181.0795, 0.6863) -> (181.3545, 0.76)
  line L3315 (181.8308, -0.865) -> (181.6295, -1.0663)
  line L3316 (181.8308, 0.485) -> (181.9045, 0.21)
  line L3317 (180.8045, -0.59) -> (180.8045, 0.21)
  line L3318 (181.6295, -1.0663) -> (181.3545, -1.14)
  line L3319 (180.8045, 0.21) -> (180.8781, 0.485)
  line L3320 (181.3545, -1.14) -> (181.0795, -1.0663)
  line L3321 (180.8781, 0.485) -> (181.0795, 0.6863)
  line L3322 (181.3545, 0.76) -> (181.6295, 0.6863)
  line L3323 (181.6295, 0.6863) -> (181.8308, 0.485)
  line L3324 (181.0795, -1.0663) -> (180.8781, -0.865)
  line L3325 (181.9045, 0.21) -> (181.9045, -0.59)
  line L3326 (180.8781, -0.865) -> (180.8045, -0.59)
  line L3327 (181.9045, -0.59) -> (181.8308, -0.865)
  arc A0 (10.5631, -8.0011) -> (8.7631, -8.0011) centre (9.6631, -8.0011) ccw
  arc A1 (8.7631, -8.0011) -> (10.5631, -8.0011) centre (9.6631, -8.0011) ccw
  arc A2 (10.5631, -5.4611) -> (8.7631, -5.4611) centre (9.6631, -5.4611) ccw
  arc A3 (8.7631, -5.4611) -> (10.5631, -5.4611) centre (9.6631, -5.4611) ccw
  arc A4 (8.7631, -2.9211) -> (10.5631, -2.9211) centre (9.6631, -2.9211) ccw
  arc A5 (10.5631, -2.9211) -> (8.7631, -2.9211) centre (9.6631, -2.9211) ccw
  line L3328 (-3.9371, -8.0011) -> (-3.9371, -8.0011)
  arc A6 (-3.9371, -8.0011) -> (-5.7371, -8.0011) centre (-4.8371, -8.0011) ccw
  arc A7 (-5.7371, -8.0011) -> (-3.9371, -8.0011) centre (-4.8371, -8.0011) ccw
  line L3329 (-3.9371, -2.9211) -> (-3.9371, -2.9211)
  arc A8 (-5.7371, -2.9211) -> (-3.9371, -2.9211) centre (-4.8371, -2.9211) ccw
  arc A9 (-3.9371, -2.9211) -> (-5.7371, -2.9211) centre (-4.8371, -2.9211) ccw
  line L3330 (3.0129, 1.189) -> (3.453, 1.1015)
  line L3331 (0.8729, 1.1015) -> (1.3129, 1.189)
  line L3332 (0.8729, -1.0235) -> (0.4998, -0.7742)
  line L3333 (3.8261, 0.8522) -> (4.0754, 0.4791)
  line L3334 (3.453, -1.0235) -> (3.0129, -1.111)
  line L3335 (1.3129, 1.189) -> (3.0129, 1.189)
  line L3336 (3.453, 1.1015) -> (3.8261, 0.8522)
  line L3337 (3.0129, -1.111) -> (1.3129, -1.111)
  line L3338 (0.4998, 0.8522) -> (0.8729, 1.1015)
  line L3339 (0.2505, 0.4791) -> (0.4998, 0.8522)
  line L3340 (0.1629, 0.039) -> (0.2505, 0.4791)
  line L3341 (4.0754, -0.4011) -> (3.8261, -0.7742)
  line L3342 (1.3129, -1.111) -> (0.8729, -1.0235)
  line L3343 (4.1629, 0.039) -> (4.0754, -0.4011)
  line L3344 (0.2505, -0.4011) -> (0.1629, 0.039)
  line L3345 (4.0754, 0.4791) -> (4.1629, 0.039)
  line L3346 (3.8261, -0.7742) -> (3.453, -1.0235)
  line L3347 (0.4998, -0.7742) -> (0.2505, -0.4011)
  line L3348 (4.0754, -11.4011) -> (3.8261, -11.7742)
  line L3349 (4.0754, -10.5209) -> (4.1629, -10.961)
  line L3350 (3.0129, -12.111) -> (1.3129, -12.111)
  line L3351 (4.1629, -10.961) -> (4.0754, -11.4011)
  line L3352 (1.3129, -9.811) -> (3.0129, -9.811)
  line L3353 (3.0129, -9.811) -> (3.453, -9.8985)
  line L3354 (1.3129, -12.111) -> (0.8729, -12.0235)
  line L3355 (0.4998, -11.7742) -> (0.2505, -11.4011)
  line L3356 (3.453, -9.8985) -> (3.8261, -10.1478)
  line L3357 (0.2505, -11.4011) -> (0.1629, -10.961)
  line L3358 (3.8261, -10.1478) -> (4.0754, -10.5209)
  line L3359 (0.8729, -12.0235) -> (0.4998, -11.7742)
  line L3360 (0.1629, -10.961) -> (0.2505, -10.5209)
  line L3361 (3.453, -12.0235) -> (3.0129, -12.111)
  line L3362 (0.4998, -10.1478) -> (0.8729, -9.8985)
  line L3363 (0.2505, -10.5209) -> (0.4998, -10.1478)
  line L3364 (0.8729, -9.8985) -> (1.3129, -9.811)
  line L3365 (3.8261, -11.7742) -> (3.453, -12.0235)
  arc A10 (195.9974, -61.2644) -> (194.7974, -61.2644) centre (195.3974, -61.2644) ccw
  arc A11 (194.7974, -61.2644) -> (195.9974, -61.2644) centre (195.3974, -61.2644) ccw
  arc A12 (192.4974, -63.5184) -> (191.2974, -63.5184) centre (191.8974, -63.5184) ccw
  arc A13 (191.2974, -63.5184) -> (192.4974, -63.5184) centre (191.8974, -63.5184) ccw
  arc A14 (175.7474, -80.3272) -> (176.9474, -80.3272) centre (176.3474, -80.3272) ccw
  arc A15 (176.9474, -80.3272) -> (175.7474, -80.3272) centre (176.3474, -80.3272) ccw
  arc A16 (173.4473, -82.5812) -> (172.2473, -82.5812) centre (172.8473, -82.5812) ccw
  arc A17 (172.2473, -82.5812) -> (173.4473, -82.5812) centre (172.8473, -82.5812) ccw
  arc A18 (175.7474, -61.2644) -> (176.9474, -61.2644) centre (176.3474, -61.2644) ccw
  arc A19 (176.9474, -61.2644) -> (175.7474, -61.2644) centre (176.3474, -61.2644) ccw
  arc A20 (172.2473, -63.5184) -> (173.4473, -63.5184) centre (172.8473, -63.5184) ccw
  arc A21 (173.4473, -63.5184) -> (172.2473, -63.5184) centre (172.8473, -63.5184) ccw
  arc A22 (175.7474, -42.2017) -> (176.9474, -42.2017) centre (176.3474, -42.2017) ccw
  arc A23 (176.9474, -42.2017) -> (175.7474, -42.2017) centre (176.3474, -42.2017) ccw
  arc A24 (172.2473, -44.4557) -> (173.4473, -44.4557) centre (172.8473, -44.4557) ccw
  arc A25 (173.4473, -44.4557) -> (172.2473, -44.4557) centre (172.8473, -44.4557) ccw
  arc A26 (175.7474, -23.1516) -> (176.9474, -23.1516) centre (176.3474, -23.1516) ccw
  arc A27 (176.9474, -23.1516) -> (175.7474, -23.1516) centre (176.3474, -23.1516) ccw
  arc A28 (172.2473, -25.4057) -> (173.4473, -25.4057) centre (172.8473, -25.4057) ccw
  arc A29 (173.4473, -25.4057) -> (172.2473, -25.4057) centre (172.8473, -25.4057) ccw
  arc A30 (157.8973, -80.3272) -> (156.6973, -80.3272) centre (157.2973, -80.3272) ccw
  arc A31 (156.6973, -80.3272) -> (157.8973, -80.3272) centre (157.2973, -80.3272) ccw
  arc A32 (154.3973, -82.5812) -> (153.1973, -82.5812) centre (153.7973, -82.5812) ccw
  arc A33 (153.1973, -82.5812) -> (154.3973, -82.5812) centre (153.7973, -82.5812) ccw
  arc A34 (156.6973, -42.2017) -> (157.8973, -42.2017) centre (157.2973, -42.2017) ccw
  arc A35 (157.8973, -42.2017) -> (156.6973, -42.2017) centre (157.2973, -42.2017) ccw
  arc A36 (154.3973, -44.4557) -> (153.1973, -44.4557) centre (153.7973, -44.4557) ccw
  arc A37 (153.1973, -44.4557) -> (154.3973, -44.4557) centre (153.7973, -44.4557) ccw
  arc A38 (157.8973, -61.2644) -> (156.6973, -61.2644) centre (157.2973, -61.2644) ccw
  arc A39 (156.6973, -61.2644) -> (157.8973, -61.2644) centre (157.2973, -61.2644) ccw
  arc A40 (153.1973, -63.5184) -> (154.3973, -63.5184) centre (153.7973, -63.5184) ccw
  arc A41 (154.3973, -63.5184) -> (153.1973, -63.5184) centre (153.7973, -63.5184) ccw
  arc A42 (156.6973, -23.1516) -> (157.8973, -23.1516) centre (157.2973, -23.1516) ccw
  arc A43 (157.8973, -23.1516) -> (156.6973, -23.1516) centre (157.2973, -23.1516) ccw
  arc A44 (154.3973, -25.4057) -> (153.1973, -25.4057) centre (153.7973, -25.4057) ccw
  arc A45 (153.1973, -25.4057) -> (154.3973, -25.4057) centre (153.7973, -25.4057) ccw
  arc A46 (137.6473, -61.2644) -> (138.8473, -61.2644) centre (138.2473, -61.2644) ccw
  arc A47 (138.8473, -61.2644) -> (137.6473, -61.2644) centre (138.2473, -61.2644) ccw
  arc A48 (134.1473, -63.5184) -> (135.3473, -63.5184) centre (134.7473, -63.5184) ccw
  arc A49 (135.3473, -63.5184) -> (134.1473, -63.5184) centre (134.7473, -63.5184) ccw
  arc A50 (138.8473, -42.2017) -> (137.6473, -42.2017) centre (138.2473, -42.2017) ccw
  arc A51 (137.6473, -42.2017) -> (138.8473, -42.2017) centre (138.2473, -42.2017) ccw
  arc A52 (134.1473, -44.4557) -> (135.3473, -44.4557) centre (134.7473, -44.4557) ccw
  arc A53 (135.3473, -44.4557) -> (134.1473, -44.4557) centre (134.7473, -44.4557) ccw
  arc A54 (138.8473, -23.1516) -> (137.6473, -23.1516) centre (138.2473, -23.1516) ccw
  arc A55 (137.6473, -23.1516) -> (138.8473, -23.1516) centre (138.2473, -23.1516) ccw
  arc A56 (134.1473, -25.4057) -> (135.3473, -25.4057) centre (134.7473, -25.4057) ccw
  arc A57 (135.3473, -25.4057) -> (134.1473, -25.4057) centre (134.7473, -25.4057) ccw
  arc A58 (137.6473, -80.3272) -> (138.8473, -80.3272) centre (138.2473, -80.3272) ccw
  arc A59 (138.8473, -80.3272) -> (137.6473, -80.3272) centre (138.2473, -80.3272) ccw
  arc A60 (134.1473, -82.5812) -> (135.3473, -82.5812) centre (134.7473, -82.5812) ccw
  arc A61 (135.3473, -82.5812) -> (134.1473, -82.5812) centre (134.7473, -82.5812) ccw
  arc A62 (119.7972, -80.3272) -> (118.5972, -80.3272) centre (119.1972, -80.3272) ccw
  arc A63 (118.5972, -80.3272) -> (119.7972, -80.3272) centre (119.1972, -80.3272) ccw
  arc A64 (115.0972, -82.5812) -> (116.2972, -82.5812) centre (115.6972, -82.5812) ccw
  arc A65 (116.2972, -82.5812) -> (115.0972, -82.5812) centre (115.6972, -82.5812) ccw
  arc A66 (119.7972, -61.2644) -> (118.5972, -61.2644) centre (119.1972, -61.2644) ccw
  arc A67 (118.5972, -61.2644) -> (119.7972, -61.2644) centre (119.1972, -61.2644) ccw
  arc A68 (115.0972, -63.5184) -> (116.2972, -63.5184) centre (115.6972, -63.5184) ccw
  arc A69 (116.2972, -63.5184) -> (115.0972, -63.5184) centre (115.6972, -63.5184) ccw
  arc A70 (118.5972, -23.1516) -> (119.7972, -23.1516) centre (119.1972, -23.1516) ccw
  arc A71 (119.7972, -23.1516) -> (118.5972, -23.1516) centre (119.1972, -23.1516) ccw
  arc A72 (116.2972, -25.4057) -> (115.0972, -25.4057) centre (115.6972, -25.4057) ccw
  arc A73 (115.0972, -25.4057) -> (116.2972, -25.4057) centre (115.6972, -25.4057) ccw
  arc A74 (119.7972, -42.2017) -> (118.5972, -42.2017) centre (119.1972, -42.2017) ccw
  arc A75 (118.5972, -42.2017) -> (119.7972, -42.2017) centre (119.1972, -42.2017) ccw
  arc A76 (115.0972, -44.4557) -> (116.2972, -44.4557) centre (115.6972, -44.4557) ccw
  arc A77 (116.2972, -44.4557) -> (115.0972, -44.4557) centre (115.6972, -44.4557) ccw
  arc A78 (99.5472, -23.1516) -> (100.7472, -23.1516) centre (100.1472, -23.1516) ccw
  arc A79 (100.7472, -23.1516) -> (99.5472, -23.1516) centre (100.1472, -23.1516) ccw
  arc A80 (97.2472, -25.4057) -> (96.0472, -25.4057) centre (96.6472, -25.4057) ccw
  arc A81 (96.0472, -25.4057) -> (97.2472, -25.4057) centre (96.6472, -25.4057) ccw
  arc A82 (99.5472, -42.2017) -> (100.7472, -42.2017) centre (100.1472, -42.2017) ccw
  arc A83 (100.7472, -42.2017) -> (99.5472, -42.2017) centre (100.1472, -42.2017) ccw
  arc A84 (97.2472, -44.4557) -> (96.0472, -44.4557) centre (96.6472, -44.4557) ccw
  arc A85 (96.0472, -44.4557) -> (97.2472, -44.4557) centre (96.6472, -44.4557) ccw
  arc A86 (100.7472, -80.3272) -> (99.5472, -80.3272) centre (100.1472, -80.3272) ccw
  arc A87 (99.5472, -80.3272) -> (100.7472, -80.3272) centre (100.1472, -80.3272) ccw
  arc A88 (96.0472, -82.5812) -> (97.2472, -82.5812) centre (96.6472, -82.5812) ccw
  arc A89 (97.2472, -82.5812) -> (96.0472, -82.5812) centre (96.6472, -82.5812) ccw
  arc A90 (100.7472, -61.2644) -> (99.5472, -61.2644) centre (100.1472, -61.2644) ccw
  arc A91 (99.5472, -61.2644) -> (100.7472, -61.2644) centre (100.1472, -61.2644) ccw
  arc A92 (96.0472, -63.5184) -> (97.2472, -63.5184) centre (96.6472, -63.5184) ccw
  arc A93 (97.2472, -63.5184) -> (96.0472, -63.5184) centre (96.6472, -63.5184) ccw
  arc A94 (195.9974, -80.3272) -> (194.7974, -80.3272) centre (195.3974, -80.3272) ccw
  arc A95 (194.7974, -80.3272) -> (195.9974, -80.3272) centre (195.3974, -80.3272) ccw
  arc A96 (191.2974, -82.5812) -> (192.4974, -82.5812) centre (191.8974, -82.5812) ccw
  arc A97 (192.4974, -82.5812) -> (191.2974, -82.5812) centre (191.8974, -82.5812) ccw
  arc A98 (195.9974, -23.1516) -> (194.7974, -23.1516) centre (195.3974, -23.1516) ccw
  arc A99 (194.7974, -23.1516) -> (195.9974, -23.1516) centre (195.3974, -23.1516) ccw
  arc A100 (192.4974, -25.4057) -> (191.2974, -25.4057) centre (191.8974, -25.4057) ccw
  arc A101 (191.2974, -25.4057) -> (192.4974, -25.4057) centre (191.8974, -25.4057) ccw
  arc A102 (80.4972, -80.3272) -> (81.6972, -80.3272) centre (81.0972, -80.3272) ccw
  arc A103 (81.6972, -80.3272) -> (80.4972, -80.3272) centre (81.0972, -80.3272) ccw
  arc A104 (78.1972, -82.5812) -> (76.9972, -82.5812) centre (77.5972, -82.5812) ccw
  arc A105 (76.9972, -82.5812) -> (78.1972, -82.5812) centre (77.5972, -82.5812) ccw
  arc A106 (81.6972, -42.2017) -> (80.4972, -42.2017) centre (81.0972, -42.2017) ccw
  arc A107 (80.4972, -42.2017) -> (81.6972, -42.2017) centre (81.0972, -42.2017) ccw
  arc A108 (76.9972, -44.4557) -> (78.1972, -44.4557) centre (77.5972, -44.4557) ccw
  arc A109 (78.1972, -44.4557) -> (76.9972, -44.4557) centre (77.5972, -44.4557) ccw
  arc A110 (81.6972, -23.1516) -> (80.4972, -23.1516) centre (81.0972, -23.1516) ccw
  arc A111 (80.4972, -23.1516) -> (81.6972, -23.1516) centre (81.0972, -23.1516) ccw
  arc A112 (76.9972, -25.4057) -> (78.1972, -25.4057) centre (77.5972, -25.4057) ccw
  arc A113 (78.1972, -25.4057) -> (76.9972, -25.4057) centre (77.5972, -25.4057) ccw
  arc A114 (81.6972, -61.2644) -> (80.4972, -61.2644) centre (81.0972, -61.2644) ccw
  arc A115 (80.4972, -61.2644) -> (81.6972, -61.2644) centre (81.0972, -61.2644) ccw
  arc A116 (78.1972, -63.5184) -> (76.9972, -63.5184) centre (77.5972, -63.5184) ccw
  arc A117 (76.9972, -63.5184) -> (78.1972, -63.5184) centre (77.5972, -63.5184) ccw
  arc A118 (62.6471, -80.3272) -> (61.4471, -80.3272) centre (62.0471, -80.3272) ccw
  arc A119 (61.4471, -80.3272) -> (62.6471, -80.3272) centre (62.0471, -80.3272) ccw
  arc A120 (57.9471, -82.5812) -> (59.1471, -82.5812) centre (58.5471, -82.5812) ccw
  arc A121 (59.1471, -82.5812) -> (57.9471, -82.5812) centre (58.5471, -82.5812) ccw
  arc A122 (62.6471, -61.2644) -> (61.4471, -61.2644) centre (62.0471, -61.2644) ccw
  arc A123 (61.4471, -61.2644) -> (62.6471, -61.2644) centre (62.0471, -61.2644) ccw
  arc A124 (57.9471, -63.5184) -> (59.1471, -63.5184) centre (58.5471, -63.5184) ccw
  arc A125 (59.1471, -63.5184) -> (57.9471, -63.5184) centre (58.5471, -63.5184) ccw
  arc A126 (61.4471, -42.2017) -> (62.6471, -42.2017) centre (62.0471, -42.2017) ccw
  arc A127 (62.6471, -42.2017) -> (61.4471, -42.2017) centre (62.0471, -42.2017) ccw
  arc A128 (59.1471, -44.4557) -> (57.9471, -44.4557) centre (58.5471, -44.4557) ccw
  arc A129 (57.9471, -44.4557) -> (59.1471, -44.4557) centre (58.5471, -44.4557) ccw
  arc A130 (42.3971, -61.2644) -> (43.5971, -61.2644) centre (42.9971, -61.2644) ccw
  arc A131 (43.5971, -61.2644) -> (42.3971, -61.2644) centre (42.9971, -61.2644) ccw